420c2cc7-42a2-4408-9224-061cd0986937 (Autodesk Fusion 360 design; units mm, degrees)
Autodesk Fusion 360 part; units mm, degrees
note: some values were not read from the file. Set by a fixed rule: which sketch regions a step uses.
sketch "Sketch1" plane through (0, 0, 0) normal (0, 1, 0) x (1, 0, 0)
  circle A0 centre (0, 0) radius 10.16
  circle A1 centre (0, 0) radius 11.43
  circle A2 centre (0, 0) radius 8.89
  circle A3 centre (0, 0) radius 9.5473
  arc A4 (11.4007, -0.8177) -> (-10.4765, -4.5704) centre (0, 0) ccw
  circle A5 centre (0, 0) radius 1.9844
  line L0 (0, 0) -> (11.43, 0) construction
  line L1 (0, 0) -> (-0.8321, -9.5109)
  line L2 (0, 0) -> (-1.6579, -9.4022)
  line L3 (0, 0) -> (-2.471, -9.222)
  line L4 (0, 0) -> (-3.2654, -8.9715)
  line L5 (0, 0) -> (-4.0349, -8.6528)
  line L6 (0, 0) -> (-4.7736, -8.2682)
  line L7 (0, 0) -> (-5.4761, -7.8207)
  line L8 (-0.8321, -9.5109) -> (-0.0021, -9.5836) construction
  line L9 (-1.6579, -9.4022) -> (-0.0169, -9.6916) construction
  line L10 (-2.471, -9.222) -> (-0.0567, -9.8689) construction
  line L11 (-3.2654, -8.9715) -> (-0.1337, -10.1113) construction
  line L12 (-4.0349, -8.6528) -> (-0.2594, -10.4133) construction
  line L13 (-4.7736, -8.2682) -> (-0.4444, -10.7677) construction
  line L14 (-5.4761, -7.8207) -> (-0.6987, -11.1658) construction
  line L15 (0, 0) -> (-6.1369, -7.3136)
  line L16 (-6.1369, -7.3136) -> (-1.031, -11.598) construction
  line L17 (0, 0) -> (-6.7509, -6.7509)
  line L18 (-6.7509, -6.7509) -> (-1.4488, -12.0531) construction
  spline S0 degree 5 poles (-1.4488, -12.0531) (-1.4353, -12.0373) (-1.4083, -12.006) (-1.3676, -11.9599) (-1.3129, -11.9) (-1.2445, -11.8272) (-1.1765, -11.7559) (-1.1098, -11.6852) (-1.045, -11.6145) (-0.9826, -11.5433) (-0.9229, -11.4713) (-0.8657, -11.3987) (-0.811, -11.3256) (-0.7585, -11.2525) (-0.7079, -11.1797) (-0.659, -11.1076) (-0.6116, -11.0362) (-0.5658, -10.9658) (-0.5217, -10.8961) (-0.4794, -10.8273) (-0.439, -10.759) (-0.4006, -10.6915) (-0.3642, -10.6246) (-0.3298, -10.5586) (-0.2973, -10.4935) (-0.2666, -10.4295) (-0.2378, -10.3668) (-0.2107, -10.3054) (-0.1853, -10.2454) (-0.1618, -10.1868) (-0.1401, -10.1297) (-0.1202, -10.0742) (-0.1021, -10.0204) (-0.0856, -9.9685) (-0.0707, -9.9189) (-0.0573, -9.8717) (-0.0453, -9.8269) (-0.0349, -9.7845) (-0.0262, -9.7446) (-0.0191, -9.7071) (-0.0137, -9.6722) (-0.0096, -9.6407) (-0.0063, -9.6132) (-0.0033, -9.5906) (-0.0005, -9.5733) (0.0016, -9.5608) (0.0022, -9.554) (0.0015, -9.5502) (0.0006, -9.5481) (0, -9.5473) knots 0 0 0 0 0 0 0.022222 0.044444 0.066667 0.088889 0.111111 0.133333 0.155556 0.177778 0.2 0.222222 0.244444 0.266667 0.288889 0.311111 0.333333 0.355556 0.377778 0.4 0.422222 0.444444 0.466667 0.488889 0.511111 0.533333 0.555556 0.577778 0.6 0.622222 0.644444 0.666667 0.688889 0.711111 0.733333 0.755556 0.777778 0.8 0.822222 0.844444 0.866667 0.888889 0.911111 0.933333 0.955556 0.977778 1 1 1 1 1 1
  line L19 (-1.5497, -12.1715) -> (-1.3478, -11.9347)
  line L20 (0.0394, -9.6047) -> (-0.0394, -9.4899)
  line L21 (-0.1514, -10.1589) -> (0, 0)
  line L22 (0, 0) -> (-0.6953, -6.1228) construction
  line L23 (0, -9.5473) -> (0, 0) construction
  spline S1 degree 5 poles (0, -9.5473) (0, -9.5025) (0, -9.4211) (0, -9.3236) (0, -9.2338) (0, -9.1496) (0, -9.072) (0, -8.9918) (0, -8.926) (0, -8.89) knots 0 0 0 0 0 0 0.2 0.4 0.6 0.8 1 1 1 1 1 1
  spline S2 degree 5 poles (-2.1407, -9.3042) (-2.1307, -9.2605) (-2.1124, -9.1812) (-2.0906, -9.0862) (-2.0704, -8.9987) (-2.0515, -8.9166) (-2.0341, -8.841) (-2.0162, -8.7629) (-2.0014, -8.6987) (-1.9933, -8.6636) knots 0 0 0 0 0 0 0.2 0.4 0.6 0.8 1 1 1 1 1 1
  line L24 (0, -9.6353) -> (0, -9.4592)
  line L25 (0, -8.9608) -> (0, -8.8192)
  line L26 (-2.1605, -9.39) -> (-2.121, -9.2184)
  line L27 (-2.0092, -8.7326) -> (-1.9775, -8.5947)
  spline S3 degree 5 poles (-1.2907, -12.0711) (-1.3003, -12.0527) (-1.3196, -12.0161) (-1.3489, -11.962) (-1.3887, -11.8914) (-1.4391, -11.8051) (-1.4893, -11.7204) (-1.5385, -11.6366) (-1.5858, -11.5531) (-1.6307, -11.4697) (-1.6728, -11.3862) (-1.7122, -11.3025) (-1.7491, -11.2191) (-1.7838, -11.1361) (-1.8168, -11.0538) (-1.8484, -10.9725) (-1.8785, -10.8924) (-1.9073, -10.8134) (-1.9347, -10.7357) (-1.9605, -10.6591) (-1.9846, -10.5835) (-2.0069, -10.5091) (-2.0273, -10.4358) (-2.046, -10.3637) (-2.0631, -10.293) (-2.0787, -10.2238) (-2.0928, -10.1561) (-2.1054, -10.0902) (-2.1166, -10.0261) (-2.1264, -9.9637) (-2.1348, -9.9032) (-2.1417, -9.8446) (-2.1473, -9.7881) (-2.1517, -9.7339) (-2.1551, -9.6822) (-2.1576, -9.6331) (-2.1592, -9.5868) (-2.1599, -9.5432) (-2.1595, -9.5023) (-2.1579, -9.4642) (-2.1553, -9.429) (-2.1523, -9.3973) (-2.1494, -9.3699) (-2.1472, -9.3472) (-2.146, -9.3296) (-2.1453, -9.317) (-2.1443, -9.3102) (-2.1429, -9.3066) (-2.1415, -9.3049) (-2.1407, -9.3042) knots 0 0 0 0 0 0 0.022222 0.044444 0.066667 0.088889 0.111111 0.133333 0.155556 0.177778 0.2 0.222222 0.244444 0.266667 0.288889 0.311111 0.333333 0.355556 0.377778 0.4 0.422222 0.444444 0.466667 0.488889 0.511111 0.533333 0.555556 0.577778 0.6 0.622222 0.644444 0.666667 0.688889 0.711111 0.733333 0.755556 0.777778 0.8 0.822222 0.844444 0.866667 0.888889 0.911111 0.933333 0.955556 0.977778 1 1 1 1 1 1
  line L28 (-1.2189, -12.2091) -> (-1.3625, -11.933)
  line L29 (-2.192, -9.3513) -> (-2.0895, -9.2571)
  point P0 (-0.1514, -10.1589)
  point P1 (0, -8.89)
  point P2 (-1.5958, -11.5338)
  point P3 (-1.8227, -11.0382)
  point P4 (-1.9812, -10.5931)
  point P5 (-2.0821, -10.2063)
  point P6 (-2.1369, -9.8839)
  point P7 (-2.1576, -9.6303)
  point P8 (-2.1566, -9.4486)
  point P9 (-2.1468, -9.34)
  point P10 (-1.9933, -8.6636)
  dimension "d2" = 22.86
  dimension "id" = 17.78
  dimension "BaseDiameter" = 19.0946
  dimension "d1" = 3.9688
  dimension "d34" = 5
  dimension "d35" = 5
  dimension "d36" = 5
  dimension "d37" = 5
  dimension "d38" = 5
  dimension "d39" = 5
  dimension "d41" = 0.8332
  dimension "d42" = 1.6663
  dimension "d43" = 2.4995
  dimension "d44" = 3.3326
  dimension "d45" = 4.1658
  dimension "d46" = 4.9989
  dimension "d47" = 5.8321
  dimension "d48" = 5
  dimension "d49" = 6.6653
  dimension "d50" = 5
  dimension "d51" = 7.4984
  dimension "d55" = 5.625
  dimension "d60" = 5
  constraint coincident A0.centre A1.centre
  constraint concentric A0 A2
  constraint coincident A1 A4.end
  constraint horizontal L0
  constraint coincident A4 L0.end
  constraint coincident A3 S0.end
  constraint coincident A3 L1.end
  constraint coincident A3 L2.end
  constraint coincident A3 L3.end
  constraint coincident A3 L4.end
  constraint coincident A3 L5.end
  constraint coincident A3 L6.end
  constraint coincident A3 L7.end
  constraint vertical A0.centre S0.end
  constraint tangent A3 L8
  constraint tangent A3 L9
  constraint tangent A3 L10
  constraint tangent A3 L11
  constraint tangent A3 L12
  constraint tangent A3 L13
  constraint tangent A3 L14
  constraint coincident A3 L15.end
  constraint tangent A3 L16
  constraint coincident A3 L17.end
  constraint tangent A3 L18
  constraint midpoint L18.end L19
  constraint midpoint S0.end L20
  constraint coincident A0 P0
  constraint coincident S0 P0
  constraint coincident P0 L21.start
  constraint coincident L23 P1
  constraint coincident A2 P1
  constraint coincident P1 S1.end
  constraint midpoint S0.end L24
  constraint midpoint P1 L25
  constraint symmetric S0.end L22 S2.start
  constraint symmetric L8.end L22 P9
  constraint symmetric L9.end L22 P8
  constraint symmetric L10.end L22 P7
  constraint symmetric L11.end L22 P6
  constraint symmetric L12.end L22 P5
  constraint symmetric L13.end L22 P4
  constraint symmetric L14.end L22 P3
  constraint symmetric L16.end L22 P2
  constraint symmetric L18.end L22 S3.start
  constraint symmetric L19.start L22 L28.start
  constraint symmetric L19.end L22 L28.end
  constraint symmetric L20.start L22 L29.start
  constraint symmetric L20.end L22 L29.end
  constraint symmetric L22 P1 P10
  constraint symmetric L22 L24.start L26.start
  constraint symmetric L22 L24.end L26.end
  constraint symmetric L22 L25.start L27.start
  constraint symmetric L22 L25.end L27.end
  constraint vertical L24
  constraint vertical L25
  measures "d2" diameter of A1
  measures "id" diameter of A2
  measures "BaseDiameter" diameter of A3
  measures "d1" diameter of A5
  measures "d34" angle of L1 L2
  measures "d35" angle of L2 L3
  measures "d36" angle of L3 L4
  measures "d37" angle of L4 L5
  measures "d38" angle of L5 L6
  measures "d39" angle of L6 L7
  measures "d41" distance of L1.end L8.end
  measures "d42" distance of L2.end L9.end
  measures "d43" distance of L3.end L10.end
  measures "d44" distance of L4.end L11.end
  measures "d45" distance of L5.end L12.end
  measures "d46" distance of L6.end L13.end
  measures "d47" distance of L7.end L14.end
  measures "d48" angle of L7 L15
  measures "d49" distance of L15.end L16.end
  measures "d50" angle of L15 L17
  measures "d51" distance of L17.end L18.end
  measures "d55" angle of L21 L22
  measures "d60" angle of L1 L23
extrude "Extrude1" add sketch "Sketch1" along normal blind 304.8 contours A0 A1 S0 S3 | A3 S0 L21 | A0 A3 L21 S3 | A2 A3 L21 S1 L24 L25 | A2 A3 L1 L21 | A2 A3 L2 S2 L26 L27 | A2 A3 L1 L2 makes body 1
pattern_circular "C-Pattern2" count 12 over 360 about axis through (0, 1.75, 0) along (0, 1, 0) of bodies 1 makes body 2 at (4.0526, 203.2, 7.9125) makes body 3 at (7.466, 203.2, 4.8261) makes body 4 at (8.8788, 203.2, 0.4466) makes body 5 at (7.8082, 203.2, -4.2502) makes body 6 at (4.8261, 203.2, -7.466) makes body 7 at (0.4466, 203.2, -8.8788) makes body 8 at (-4.0526, 203.2, -7.9125) makes body 9 at (-7.466, 203.2, -4.8261) makes body 10 at (-8.8788, 203.2, -0.4466) makes body 11 at (-7.9125, 203.2, 4.0526) makes body 12 at (-4.8261, 203.2, 7.466)
extrude "Extrude2" add sketch "Sketch1" along normal blind 304.8 contours A2 A5 L17 L21 | A2 A5 L1 L21 | A2 A5 L1 L2 | A2 A5 L2 L3 | A2 A5 L3 L4 | A2 A5 L15 L17 | A2 A5 L4 L5 | A2 A5 L7 L15 | A2 A5 L5 L6 | A2 A5 L6 L7 bodies 1 2 3 4 5 6 7 8 9 10 11 12
ref_plane "WorkPlane1" through (6.2747, 152.4, -0.8261) normal (0.130526, 0, 0.991445) x (0.991445, 0, -0.130526)
fillet "Fillet1" [suppressed]
mirror "Mirror3" [suppressed]
pattern_circular "C-Pattern1" [suppressed]
equation "d = 0.8 in"
equation "OutsideDiameter = d2"
equation "PitchDiameter = d"
equation "id = PitchDiameter - 2 * ( PitchDiameter / TeethNumber )"
equation "BaseDiameter = PitchDiameter * cos(20 deg)"
equation "Length = 12 in"
equation "t = 16"
equation "ShaftDiameter = d1"
equation "TeethNumber = t"
equation "Pitch = 32"
equation "d30 = ( 1.25 * ( PitchDiameter / TeethNumber ) ) - ( PitchDiameter / TeethNumber )"
equation "Basecircum = PI * PitchDiameter * cos(20 deg)"
equation "d41 = Basecircum * 5 / 360"
equation "d42 = Basecircum * 10 / 360"
equation "d43 = Basecircum * 15 / 360"
equation "d44 = Basecircum * 20 / 360"
equation "d45 = Basecircum * 25 / 360"
equation "d46 = Basecircum * 30 / 360"
equation "d47 = Basecircum * 35 / 360"
equation "d49 = Basecircum * 40 / 360"
equation "d51 = Basecircum * 45 / 360"
equation "d55 = ( 360 / ( 4 * TeethNumber ) ) * 1 deg"
